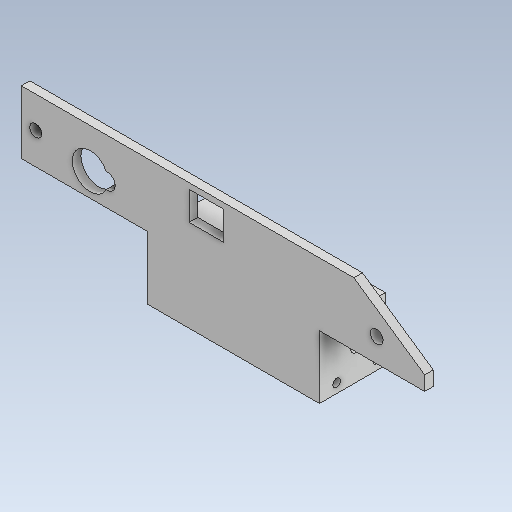
# Autodesk Inventor part: wheel-adapter
Saved by Autodesk Inventor 2020 (Build 240168000, 168)
## iProperties
Created: 2020-05-05
Part Number: wheel-adapter
Material: Ogólny
Document SubType Name: Modeling
Designer: blep
Density: 1 g/cm^3
Appearance: Domyślna
Author: blep
Autodesk Inventor part; units mm, degrees
ref_plane "YZ Plane" through (0, 0, 0) normal (1, 0, 0) x (0, 1, 0)
ref_plane "XZ Plane" through (0, 0, 0) normal (0, 1, 0) x (-1, 0, 0)
ref_plane "XY Plane" through (0, 0, 0) normal (0, 0, 1) x (1, 0, 0)
sketch "Szkic1" plane through (0, 0, 0) normal (0, 0, 1) x (1, 0, 0)
  line L0 (-106, 20) -> (0, 20) projected
  line L1 (-106, 20) -> (-106, -2) projected
  line L2 (-106, -2) -> (24.7184, -2) projected
  line L3 (24.7184, -2) -> (24.7184, 3) projected
  line L4 (24.7184, 3) -> (0, 20) projected
  circle A0 centre (8, 6.2) radius 2 construction
  circle A1 centre (8, 6.2) radius 2.25
  line L5 (-57.5, 18) -> (-45.5, 18)
  line L6 (-45.5, 18) -> (-45.5, 8)
  line L7 (-45.5, 8) -> (-57.5, 8)
  line L8 (-57.5, 8) -> (-57.5, 18)
  line L9 (-70, 12.4) -> (-70, 0) construction
  arc A2 (-86.6773, 8.9692) -> (-86.6773, 3.4308) centre (-92, 6.2) ccw construction
  arc A3 (-86, 3.7) -> (-86, 8.7) centre (-86, 6.2) ccw construction
  arc A4 (-86.2337, 3.7) -> (-86.6773, 3.4308) centre (-86.2337, 3.2) ccw construction
  line L10 (-86.2337, 3.7) -> (-86, 3.7) construction
  arc A5 (-86.6773, 8.9692) -> (-86.2337, 8.7) centre (-86.2337, 9.2) ccw construction
  line L11 (-86, 8.7) -> (-86.2337, 8.7) construction
  arc A6 (-86.375, 8.9243) -> (-86.375, 3.4757) centre (-92, 6.2) ccw
  arc A7 (-86.375, 3.4757) -> (-86.375, 8.9243) centre (-86, 6.2) ccw
  line L12 (-116, 20) -> (-106, 20)
  line L13 (-106, 20) -> (-106, -2)
  line L14 (-106, -2) -> (-116, -2)
  line L15 (-116, -2) -> (-116, 20)
  line L16 (-92, 6.2) -> (-92, -8.9) construction
  line L17 (-92, -8.9) -> (-1, -8.9) construction
  line L18 (-72, -24) -> (-12, -24)
  line L19 (-12, -24) -> (-12, -2)
  line L20 (-12, -2) -> (-72, -2)
  line L21 (-72, -2) -> (-72, -24)
  point P0 (0, 0)
  point P1 (-7.9, -2)
  point P2 (-12, -2)
  dimension "d0" = 0.25
  dimension "d1" = 12.5
  dimension "d2" = 12
  dimension "d3" = 2
  dimension "d4" = 10
  dimension "d5" = 0.25
  dimension "d6" = 10
  dimension "d11" = 91
  dimension "d14" = 20
  dimension "d15" = 20
  constraints: 28 end point, 7 parallel, 4 collinear, 4 perpendicular, 4 point on circle, 3 centre point, 3 horizontal, 1 point on line, 1 vertical, 1 other
  measures "d0" radial gap between concentric circles of A0 A1
  measures "d1" distance between parallel lines of L9 L8
  measures "d2" distance of L5.start L5.end
  measures "d3" distance between parallel lines of L0 L5
  measures "d4" distance of L5.end L6.end
  measures "d5" radial gap between concentric circles of A6 A2
  measures "d6" distance between parallel lines of L15 L1
  measures "d11" distance of L16.end L17.end
  measures "d14" distance from line of L21 L16.start
  measures "d15" distance from line of L19 A0.centre
extrude "Wyciągnięcie proste1" add sketch "Szkic1" along normal blind 3
sketch "Szkic2" plane through (0, 0, 0) normal (0, 0, -1) x (-1, 0, 0)
  line L0 (12, -2) -> (18, -2)
  line L1 (18, -2) -> (18, -24)
  line L2 (18, -24) -> (12, -24)
  line L3 (12, -24) -> (12, -2)
  line L4 (66, -2) -> (72, -2)
  line L5 (72, -2) -> (72, -24)
  line L6 (72, -24) -> (66, -24)
  line L7 (66, -24) -> (66, -2)
  line L8 (72, -2) -> (72, -24) projected
  line L9 (12, -24) -> (12, -2) projected
  line L10 (72, -24) -> (12, -24) projected
  point P0 (0, 0)
  dimension "d16" = 6
  dimension "d17" = 6
  constraints: 16 end point, 6 collinear, 4 parallel, 2 horizontal, 2 perpendicular
  measures "d16" distance between parallel lines of L3 L1
  measures "d17" distance between parallel lines of L5 L7
extrude "Wyciągnięcie proste2" add sketch "Szkic2" along normal blind 20
sketch "Szkic4" plane through (-66, -24, 0) normal (1, 0, 0) x (0, 0, -1)
  line L0 (3, 18.7) -> (17, 18.7) construction
  line L1 (17, 18.7) -> (17, 3.3) construction
  line L2 (17, 3.3) -> (3, 3.3) construction
  line L3 (3, 3.3) -> (3, 18.7) construction
  line L4 (3, 18.7) -> (10, 11) construction
  line L5 (10, 11) -> (3, 3.3) construction
  line L6 (17, 3.3) -> (10, 11) construction
  line L7 (0, 22) -> (20, 22) construction
  line L8 (3, 18.7) -> (0, 22) construction
  line L9 (0, 0) -> (20, 0) construction
  line L10 (17, 3.3) -> (20, 0) construction
  line L11 (3, 3.3) -> (0, 0) construction
  line L12 (20, 22) -> (20, 0) construction
  point P0 (0, 24)
  dimension "d20" = 3
  constraints: 20 end point, 5 coincident, 4 equal length, 2 parallel, 1 collinear, 1 horizontal, 1 perpendicular
  measures "d20" distance between parallel lines of L12 L1
hole "Otwór2" at (-66, -13, -10) direction (-1, 0, 0) diameter 4.25 end through all both
sketch "Szkic5" plane through (-18, -24, 0) normal (-1, 0, 0) x (0, 0, 1)
  line L0 (-13.5, 11) -> (-13.5, 8.9793) projected
  line L1 (-13.5, 13.0207) -> (-13.5, 11) projected
  line L2 (-13.5, 8.9793) -> (-11.75, 7.9689) projected
  line L3 (-11.75, 7.9689) -> (-10, 6.9585) projected
  line L4 (-10, 6.9585) -> (-8.25, 7.9689) projected
  line L5 (-8.25, 7.9689) -> (-6.5, 8.9793) projected
  line L6 (-6.5, 8.9793) -> (-6.5, 11) projected
  line L7 (-6.5, 11) -> (-6.5, 13.0207) projected
  line L8 (-6.5, 13.0207) -> (-8.25, 14.0311) projected
  line L9 (-8.25, 14.0311) -> (-10, 15.0415) projected
  line L10 (-10, 15.0415) -> (-11.75, 14.0311) projected
  line L11 (-11.75, 14.0311) -> (-13.5, 13.0207) projected
  line L12 (-14, 8.6906) -> (-14, 11)
  line L13 (-14, 11) -> (-14, 13.3094)
  line L14 (-14, 13.3094) -> (-12, 14.4641)
  line L15 (-12, 14.4641) -> (-10, 15.6188)
  line L16 (-10, 15.6188) -> (-8, 14.4641)
  line L17 (-8, 14.4641) -> (-6, 13.3094)
  line L18 (-6, 13.3094) -> (-6, 11)
  line L19 (-6, 11) -> (-6, 8.6906)
  line L20 (-6, 8.6906) -> (-8, 7.5359)
  line L21 (-8, 7.5359) -> (-10, 6.3812)
  line L22 (-10, 6.3812) -> (-12, 7.5359)
  line L23 (-12, 7.5359) -> (-14, 8.6906)
  point P0 (0, 24)
  dimension "d36" = 0.5
  constraints: 24 end point, 11 other
  measures "d36" distance between parallel lines of L0 L12
extrude "Wyciągnięcie proste3" cut sketch "Szkic5" against normal blind 3 contours L1 L11 L10 L9 L8 L7 L6 L5 L4 L3 L2 L0 | L12 L13 L14 L15 L16 L17 L18 L19 L20 L21 L22 L23
sketch "Szkic6" plane through (-66, -24, 0) normal (1, 0, 0) x (0, 0, -1)
  line L0 (14, 8.6906) -> (14, 13.3094) projected
  line L1 (14, 13.3094) -> (10, 15.6188) projected
  line L2 (10, 15.6188) -> (6, 13.3094) projected
  line L3 (6, 13.3094) -> (6, 8.6906) projected
  line L4 (6, 8.6906) -> (10, 6.3812) projected
  line L5 (10, 6.3812) -> (14, 8.6906) projected
  point P0 (0, 24)
extrude "Wyciągnięcie proste4" cut sketch "Szkic6" against normal blind 3
sketch "Szkic7" plane through (0, 0, 3) normal (0, 0, 1) x (1, 0, 0)
  line L0 (-116, 20) -> (-116, -2) projected
  line L1 (-116, 20) -> (-106, 20) projected
  line L2 (-106, -2) -> (-116, -2) projected
  line L3 (-106, 20) -> (-106, -2) projected
  line L4 (0, 20) -> (-116, 20) construction
  line L5 (-116, 20) -> (-111, 9) construction
  line L6 (-111, 9) -> (-106, -2) construction
  line L7 (-116, -2) -> (-72, -2) construction
  line L8 (-116, -2) -> (-111, 9) construction
  point P0 (0, 0)
  constraints: 6 end point, 2 equal length, 1 coincident
hole "Otwór3" at (-111, 9, 3) direction (0, 0, -1) diameter 4.25 end through all
sketch "Szkic8" plane through (0, 0, 0) normal (0, 0, -1) x (-1, 0, 0)
  line L0 (66, -18) -> (18, -18)
  line L1 (18, -18) -> (18, -24)
  line L2 (18, -24) -> (66, -24)
  line L3 (66, -24) -> (66, -18)
  line L4 (66, -2) -> (18, -2)
  line L5 (18, -2) -> (18, -8)
  line L6 (18, -8) -> (66, -8)
  line L7 (66, -8) -> (66, -2)
  line L8 (66, -24) -> (18, -24) projected
  point P0 (0, 0)
  dimension "d48" = 6
  dimension "d49" = 6
  constraints: 16 end point, 4 parallel, 2 coincident, 2 horizontal, 2 perpendicular, 1 collinear, 1 point on line
  measures "d48" distance between parallel lines of L2 L0
  measures "d49" distance between parallel lines of L4 L6
extrude "Wyciągnięcie proste5" add sketch "Szkic8" along normal blind 20
hole "Otwór1" at (-66, -5.3, -3) at (-66, -20.7, -17) at (-66, -20.7, -3) at (-66, -5.3, -17) direction (-1, 0, 0) diameter 2.75 end through all both
equation "\"d15\" = d14"
equation "\"d17\" = d16"
equation "\"d49\" = d48"
